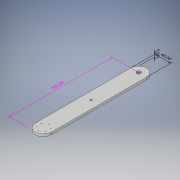
# Autodesk Inventor part: GroundArm
Saved by Autodesk Inventor 2019 (Build 230136000, 136)
## iProperties
Created: 2018-06-10
Part Number: GroundArm
Material: Ogólny
Document SubType Name: Modeling
Designer: Kamil
Density: 1 g/cm^3
Appearance: Domyślna
Author: Kamil
## iProperties of the stored document GroundArm_Drukowanie 3D.ipt
Created: 2018-06-24
Part Number: GroundArm_Drukowanie 3D
Material: Ogólny
Document SubType Name: Modeling
Designer: Kamil
Density: 1 g/cm^3
Appearance: Domyślna
Author: Kamil
Autodesk Inventor part; units mm, degrees
ref_plane "YZ Plane" through (0, 0, 0) normal (1, 0, 0) x (0, 1, 0)
ref_plane "XZ Plane" through (0, 0, 0) normal (0, 1, 0) x (-1, 0, 0)
ref_plane "XY Plane" through (0, 0, 0) normal (0, 0, 1) x (1, 0, 0)
sketch "Szkic1" plane through (0, 0, 0) normal (0, 1, 0) x (-1, 0, 0)
  line L0 (-20, 140) -> (20, 140)
  line L1 (20, 140) -> (20, -120)
  line L2 (0, -140) -> (0, -140)
  line L3 (-20, -120) -> (-20, 140)
  arc A0 (0, -140) -> (20, -120) centre (0, -120) ccw
  arc A1 (-20, -120) -> (0, -140) centre (0, -120) ccw
  circle A2 centre (0, -120) radius 5
  circle A3 centre (0, 0) radius 2.5
  point P0 (20, -120)
  point P1 (0, -140)
  point P2 (-20, -120)
  point P3 (20, -120)
  point P4 (-20, -120)
  point P5 (0, -140)
  dimension "d3" = 20
  dimension "d4" = 20
  dimension "d9" = 5
  constraints: 8 end point, 5 coincident, 4 centre point, 4 point on circle, 4 tangent, 2 parallel, 2 point on line, 1 horizontal, 1 midpoint, 1 perpendicular
  measures "d3" radius of A0
  measures "d4" radius of A1
  measures "d9" diameter of A3
extrude "Wyciągnięcie proste2" add sketch "Szkic1" along normal blind 6
sketch "Szkic2" plane through (0, 6, 0) normal (0, 1, 0) x (1, 0, 0)
  line L0 (0, -106.7) -> (11.5181, -113.35)
  line L1 (11.5181, -113.35) -> (11.5181, -126.65)
  line L2 (11.5181, -126.65) -> (0, -133.3)
  line L3 (0, -133.3) -> (-11.5181, -126.65)
  line L4 (-11.5181, -126.65) -> (-11.5181, -113.35)
  line L5 (-11.5181, -113.35) -> (0, -106.7)
  circle A0 centre (-11.5181, -113.35) radius 0.75
  circle A1 centre (0, -106.7) radius 0.75
  circle A2 centre (11.5181, -113.35) radius 0.75
  circle A3 centre (11.5181, -126.65) radius 0.75
  circle A4 centre (0, -133.3) radius 0.75
  circle A5 centre (-11.5181, -126.65) radius 0.75
  point P0 (0, 0)
  point P1 (-20.5841, -116.7396)
  point P2 (0, -120)
  point P3 (0, -120)
  point P4 (0, -120)
  dimension "d12" = 1.5
  dimension "d13" = 1.5
  dimension "d14" = 1.5
  dimension "d15" = 1.5
  dimension "d16" = 1.5
  dimension "d17" = 1.5
  constraints: 12 end point, 8 coincident, 6 centre point, 13 other
  measures "d12" diameter of A0
  measures "d13" diameter of A1
  measures "d14" diameter of A2
  measures "d15" diameter of A3
  measures "d16" diameter of A4
  measures "d17" diameter of A5
extrude "Wyciągnięcie proste3" cut sketch "Szkic2" against normal blind 6 contours L5 A1 L0 | L0 A1 L5 | A2 L1 L0 | L0 L1 A2 | A0 L4 L5 | L5 L4 A0 | A3 L2 L1 | L1 L2 A3 | A5 L3 L4 | L4 L3 A5 | A4 L3 L2 | L2 L3 A4
sketch "Szkic3" plane through (0, 0, 0) normal (0, -1, 0) x (1, 0, 0)
  circle A0 centre (0, -120) radius 5
  circle A1 centre (0, -120) radius 2.5
  point P0 (0, 0)
  dimension "d30" = 10
  dimension "d31" = 5
  constraints: 2 centre point, 1 coincident
  measures "d30" diameter of A0
  measures "d31" diameter of A1
extrude "Wyciągnięcie proste4" add sketch "Szkic3" against normal blind 2
fillet "Zaokrąglenie1" radius 20 1 edges at (20, 3, 140)
fillet "Zaokrąglenie2" radius 20 1 edges at (-20, 3, 140)
